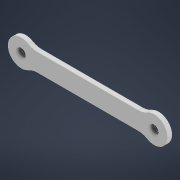
# Autodesk Inventor part: Рычаг_1
Saved by Autodesk Inventor 2021.2 (Build 252289000, 289)
## iProperties
Created: 2021-05-30
Part Number: Рычаг_1
Material: Типовые
Document SubType Name: Modeling
Designer: Admin
Density: 1 g/cm^3
Appearance: По умолчанию
Mass: 1443.25 g
Surface Area: 1850.44 cm^2
Volume: 1443.25 cm^3
Author: Admin
Autodesk Inventor part; units mm, degrees
ref_plane "YZ Plane" through (0, 0, 0) normal (1, 0, 0) x (0, 1, 0)
ref_plane "XZ Plane" through (0, 0, 0) normal (0, 1, 0) x (-1, 0, 0)
ref_plane "XY Plane" through (0, 0, 0) normal (0, 0, 1) x (1, 0, 0)
sketch "Эскиз1" plane through (0, 0, 0) normal (0, 0, 1) x (1, 0, 0)
  arc A0 (7.7262, 12.8571) -> (7.7262, -12.8571) centre (0, 0) ccw
  line L0 (18.0278, 10) -> (131.9722, 10)
  line L1 (18.0278, -10) -> (131.9722, -10)
  arc A1 (142.2738, -12.8571) -> (142.2738, 12.8571) centre (150, 0) ccw
  arc A2 (7.7262, 12.8571) -> (18.0278, 10) centre (18.0278, 30) ccw
  arc A3 (18.0278, -10) -> (7.7262, -12.8571) centre (18.0278, -30) ccw
  arc A4 (142.2738, -12.8571) -> (131.9722, -10) centre (131.9722, -30) ccw
  arc A5 (131.9722, 10) -> (142.2738, 12.8571) centre (131.9722, 30) ccw
  point P0 (11.1803, 10)
  point P1 (138.8197, 10)
  point P2 (11.1803, -10)
  point P3 (138.8197, -10)
  dimension "d0" = 30
  dimension "d1" = 30
  dimension "d5" = 150
  dimension "d17" = 20
  dimension "d18" = 20
  constraints: 16 point on circle, 8 tangent, 6 centre point, 4 end point, 4 point on line, 3 equal radius, 2 vertical alignment, 1 coincident, 1 horizontal alignment
  measures "d0" diameter of A0
  measures "d1" diameter of A1
  measures "d5" distance of point (0, 0) A1.centre
  measures "d17" distance between parallel lines of L1 L0
  measures "d18" radius of A2
extrude "Выдавливание1" add sketch "Эскиз1" along normal blind 5
sketch "Эскиз2" plane through (0, 0, 5) normal (0, 0, 1) x (1, 0, 0)
  arc A0 (142.2738, -12.8571) -> (142.2738, 12.8571) centre (150, 0) ccw projected
  point P0 (0, 0)
  point P1 (0, 0)
  point P2 (88.8197, -10)
  point P3 (88.8197, 10)
  constraints: 2 coincident
hole "Отверстие1" at (0, 0, 5) at (150, 0, 5) direction (0, 0, -1) diameter 10 end through all
